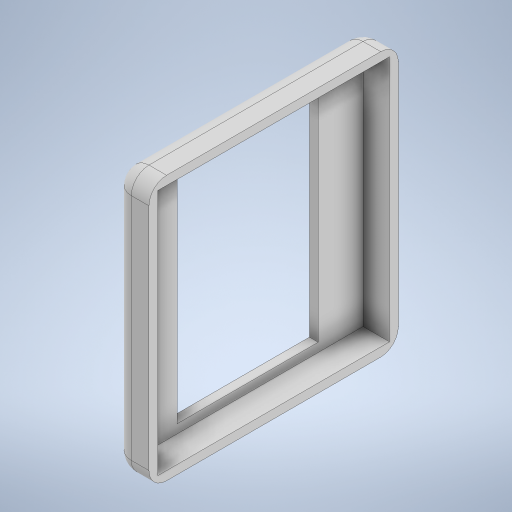
# Autodesk Inventor part: outer_casing
Saved by Autodesk Inventor 2023 (Build 270158000, 158)
## iProperties
Created: 2023-02-11
Part Number: outer_casing
Material: Generic
Document SubType Name: Modeling
Designer: Lauren
Density: 1 g/cm^3
Appearance: Default
Author: Lauren
Autodesk Inventor part; units mm, degrees
ref_plane "YZ Plane" through (0, 0, 0) normal (1, 0, 0) x (0, 1, 0)
ref_plane "XZ Plane" through (0, 0, 0) normal (0, 1, 0) x (-1, 0, 0)
ref_plane "XY Plane" through (0, 0, 0) normal (0, 0, 1) x (1, 0, 0)
sketch "Sketch1" plane through (0, 0, 0) normal (1, 0, 0) x (0, 1, 0)
  line L0 (0, 0) -> (190.5, 0)
  line L1 (190.5, 0) -> (190.5, -179.6034)
  line L2 (190.5, -179.6034) -> (0, -179.6034)
  line L3 (0, -179.6034) -> (0, 0)
  dimension "d0" = 190.5
  dimension "d1" = 179.6034
  constraints: 8 end point, 2 parallel, 1 horizontal, 1 perpendicular
  measures "d0" distance of L1.end L2.end
  measures "d1" distance of L0.end L1.end
extrude "Extrusion1" add sketch "Sketch1" along normal blind 25.4
shell "Shell1" thickness 6.35 removed faces 1 at (25.4, 127, -119.7356)
sketch "Sketch2" plane through (6.35, 6.35, -173.2534) normal (1, 0, 0) x (0, 0, -1)
  line L0 (-32.2834, 171.45) -> (-133.8834, 171.45)
  line L1 (-133.8834, 171.45) -> (-133.8834, 6.35)
  line L2 (-133.8834, 6.35) -> (-32.2834, 6.35)
  line L3 (-32.2834, 6.35) -> (-32.2834, 171.45)
  line L4 (-166.9034, 177.8) -> (0, 177.8) projected
  line L5 (-166.9034, 0) -> (-166.9034, 177.8) projected
  point P0 (-173.2534, -6.35)
  dimension "d5" = 165.1
  dimension "d6" = 101.6
  dimension "d7" = 6.35
  dimension "d8" = 33.02
  constraints: 8 end point, 2 parallel, 1 horizontal, 1 perpendicular
  measures "d5" distance of L0.end L1.end
  measures "d6" distance of L1.end L2.end
  measures "d7" distance between parallel lines of L4 L0
  measures "d8" distance between parallel lines of L5 L1
extrude "Extrusion2" cut sketch "Sketch2" against normal through all
fillet "Fillet1" radius 12.7 1 edges at (12.7, 190.5, -179.6034)
fillet "Fillet2" radius 12.7 8 edges at (12.7, 190.5, 0) (12.7, 0, 0) (12.7, 0, -179.6034) (0, 0, -89.8017) (0, 186.7803, -175.8837) (0, 190.5, -83.4517) (0, 88.9, -179.6034) (0, 95.25, 0)
body "Solid1"
